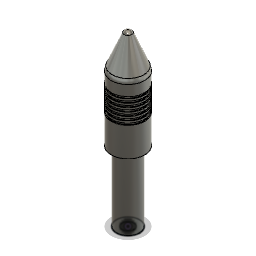
ideal-61-312-multimeter-probe-cap-v10 (Autodesk Fusion 360 design; units mm, degrees)
Autodesk Fusion 360 part; units mm, degrees
sketch "Sketch1" plane through (0, 0, 0) normal (0, 1, 0) x (1, 0, 0)
  circle A0 centre (0, 0) radius 1.2
  circle A1 centre (0, 0) radius 2.4
  dimension "d1" = 2.4
  dimension "d2" = 1.2
  constraint coincident A0.centre A1.centre
  measures "d1" diameter of A0
  measures "d2" distance of A0
extrude "Extrude1" add sketch "Sketch1" along normal blind 13.5
sketch "Sketch2" plane through (0, 13.5, 0) normal (0, 1, 0) x (-1, 0, 0)
  circle A0 centre (0, 0) radius 1.2
  circle A1 centre (0, 0) radius 2.4
  circle A2 centre (0, 0) radius 1.2
  circle A3 centre (0, 0) radius 2.4
extrude "Extrude2" add sketch "Sketch2" along normal blind 1.2 contours A0 A2 | A1 A3
sketch "Sketch3" plane through (0, 14.7, 0) normal (0, 1, 0) x (-1, 0, 0)
  circle A0 centre (0, 0) radius 2.4
  circle A1 centre (0, 0) radius 3.5
  dimension "d11" = 7
  constraint concentric A0 A1
  measures "d11" diameter of A1
extrude "Extrude3" add sketch "Sketch3" along normal blind 14 contours A0 | A1
extrude "Extrude4" add 1 faces at (0.7915, 28.7, 0.6312) along direction (0, 1, 0) blind 7 draft -22.5
fillet "Fillet1" radius 0.8 1 faces at (-0.4122, 35.7, -0.15)
fillet "Fillet2" radius 2.5 1 edges at (3.2631, 28.7, -1.2657)
sketch "Sketch4" plane through (0, 14.7, 0) normal (0, -1, 0) x (1, 0, 0)
  circle A0 centre (0, 0) radius 3.5
  circle A1 centre (0, 0) radius 2.4
sketch "Sketch5" plane through (0, 0, 0) normal (0, 1, 0) x (1, 0, 0)
  circle A0 centre (0, 0) radius 3.5
  circle A1 centre (0, 0) radius 3.3
  dimension "d20" = 7
  dimension "d21" = 6.6
  constraint coincident A0.centre A1.centre
  measures "d20" diameter of A0
  measures "d21" diameter of A1
extrude "Extrude7" cut sketch "Sketch5" along normal blind 20.8 and the other way blind -21.2
extrude "Extrude8" cut sketch "Sketch5" along normal blind 21.6 and the other way blind -22
extrude "Extrude9" cut sketch "Sketch5" along normal blind 22.4 and the other way blind -22.8
extrude "Extrude10" cut sketch "Sketch5" along normal blind 23.2 and the other way blind -23.6
extrude "Extrude11" cut sketch "Sketch5" along normal blind 24 and the other way blind -24.4
extrude "Extrude12" cut sketch "Sketch5" along normal blind 24.8 and the other way blind -25.2
extrude "Extrude13" cut sketch "Sketch5" along normal blind 25.6 and the other way blind -26
extrude "Extrude15" cut sketch "Sketch1" along normal blind 32.4 contours A0
equation "d1 = ProbeDiameter + ProbeDeiameterClearence"
equation "d2 = WallThickness"
equation "d3 = ProbeLenght"
equation "d5 = WallThickness"
equation "ProbeDiameter = 2.4 mm"
equation "ProbeDeiameterClearence = 0 mm"
equation "ProbeLenght = 13.5 mm"
equation "WallThickness = 1.2 mm"
equation "RidgeBaseDist = 19.6 mm"
equation "RidgeDistIncrement = 0.4 mm"
equation "RidgeSecondDist = -19.2 mm"
equation "RidgeCutGap = -0.4 mm"
equation "d34 = RidgeBaseDist + ( 3 * RidgeDistIncrement )"
equation "d36 = RidgeSecondDist + ( 5 * RidgeCutGap )"
equation "d38 = RidgeBaseDist + ( 5 * RidgeDistIncrement )"
equation "d40 = RidgeSecondDist + ( 7 * RidgeCutGap )"
equation "d42 = RidgeBaseDist + ( 7 * RidgeDistIncrement )"
equation "d44 = RidgeSecondDist + ( 9 * RidgeCutGap )"
equation "d46 = RidgeBaseDist + ( 9 * RidgeDistIncrement )"
equation "d48 = RidgeSecondDist + ( 11 * RidgeCutGap )"
equation "d50 = RidgeBaseDist + ( 11 * RidgeDistIncrement )"
equation "d52 = RidgeSecondDist + ( 13 * RidgeCutGap )"
equation "d54 = RidgeBaseDist + ( 13 * RidgeDistIncrement )"
equation "d56 = RidgeSecondDist + ( 15 * RidgeCutGap )"
equation "d58 = RidgeBaseDist + ( 15 * RidgeDistIncrement )"
equation "d60 = RidgeSecondDist + ( 17 * RidgeCutGap )"
